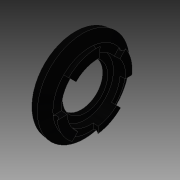
# Autodesk Inventor part: rope_pulley
Saved by Autodesk Inventor 2014 (Build 180170000, 170)
## iProperties
Created: 2013-12-08
Part Number: rope_pulley
Material: ABS Plastic
Document SubType Name: Modeling
Designer: buben
Density: 1.06 g/cm^3
Appearance: Anodized - Black
d0: 45,00 deg
d1: 1,000 mm
d2: 3,000 mm
d4: 6,000 mm
d5: 2,000 mm
d8: 7,000 mm
d9: 17,000 mm
d10: 22,000 mm
d12: 4,000 ul
d14: 135,00 deg
d16: 4,424 mm
d17: 0,00 deg
d18: 2,424 mm
d19: 0,00 deg
d20: 1,000 mm
Author: buben
Autodesk Inventor part; units mm, degrees
ref_plane "YZ Plane" through (0, 0, 0) normal (1, 0, 0) x (0, 1, 0)
ref_plane "XZ Plane" through (0, 0, 0) normal (0, 1, 0) x (-1, 0, 0)
ref_plane "XY Plane" through (0, 0, 0) normal (0, 0, 1) x (1, 0, 0)
sketch "Sketch1" plane through (0, 0, 0) normal (0, 0, 1) x (1, 0, 0)
  line L0 (3.175, 17) -> (4.5761, 13.6173)
  line L1 (6.4239, 13.6173) -> (7.825, 17)
  arc A0 (4.5761, 13.6173) -> (6.4239, 13.6173) centre (5.5, 14) ccw
  line L2 (7.825, 17) -> (9, 17)
  line L3 (3.175, 17) -> (0, 17)
  line L4 (2, 11) -> (9, 11)
  line L5 (9, 17) -> (9, 11)
  line L6 (0, 17) -> (0, 8.5)
  line L7 (2, 11) -> (2, 8.5)
  line L8 (2, 8.5) -> (0, 8.5)
  line L9 (0, 0) -> (2, 0) construction
  point P0 (5.5, 11)
  dimension "d0" = 45
  dimension "d1" = 1
  dimension "d2" = 3
  dimension "d4" = 6
  dimension "d5" = 2
  dimension "d8" = 7
  dimension "d9" = 17
  dimension "d10" = 22
  constraints: 20 end point, 4 parallel, 4 vertical alignment, 2 perpendicular, 2 point on circle, 2 tangent, 1 centre point, 1 coincident, 1 collinear, 1 equal length, 1 horizontal, 1 horizontal alignment, 1 midpoint
  measures "d0" angle of L1 L0
  measures "d1" radius of A0
  measures "d2" vertical distance of L0.start A0.centre
  measures "d4" distance of L4.end L2.end
  measures "d5" distance of L7.end L6.end
  measures "d8" distance of L4.start L4.end
  measures "d9" diameter of L8 L9
  measures "d10" diameter of L4 L9
revolve "Revolution1" add sketch "Sketch1" angle 360 about axis through (0, 0, 0) along (1, 0, 0)
sketch "Sketch2" plane through (9, 0, 0) normal (1, 0, 0) x (0, 0, -1)
  circle A0 centre (0, 0) radius 11 projected
  circle A1 centre (0, 0) radius 17 projected
  line L0 (-17, 0) -> (17, 0) construction
  line L1 (-12.0208, -12.0208) -> (12.0208, 12.0208) construction
  line L2 (0, -17) -> (0, 17) construction
  line L3 (12.0208, -12.0208) -> (-12.0208, 12.0208) construction
  line L4 (-17, 0) -> (-11, 0)
  line L5 (-7.7782, 7.7782) -> (-12.0208, 12.0208)
  line L6 (0, 17) -> (0, 11)
  line L7 (12.0208, 12.0208) -> (7.7782, 7.7782)
  line L8 (11, 0) -> (17, 0)
  line L9 (12.0208, -12.0208) -> (7.7782, -7.7782)
  line L10 (0, -17) -> (0, -11)
  line L11 (-7.7782, -7.7782) -> (-12.0208, -12.0208)
  arc A2 (7.7782, 7.7782) -> (0, 11) centre (0, 0) ccw
  arc A3 (12.0208, 12.0208) -> (0, 17) centre (0, 0) ccw
  arc A4 (7.7782, -7.7782) -> (11, 0) centre (0, 0) ccw
  arc A5 (12.0208, -12.0208) -> (17, 0) centre (0, 0) ccw
  arc A6 (-12.0208, 12.0208) -> (-17, 0) centre (0, 0) ccw
  arc A7 (-12.0208, -12.0208) -> (0, -17) centre (0, 0) ccw
  arc A8 (-7.7782, 7.7782) -> (-11, 0) centre (0, 0) ccw
  arc A9 (-7.7782, -7.7782) -> (0, -11) centre (0, 0) ccw
  dimension "d14" = 135
  constraints: 25 end point, 18 point on circle, 8 centre point, 8 point on line, 4 concentric, 4 midpoint, 3 coincident, 2 collinear, 1 horizontal, 12 other
extrude "Extrusion1" cut sketch "Sketch2" against normal blind 4.424 contours L8 A1 L9 A0 | A0 L6 A1 L7 | L10 A1 L11 A0 | A0 L4 A1 L5
sketch "Sketch3" plane through (9, 0, 17) normal (1, 0, 0) x (0, 0, -1)
  line L0 (4.9792, -12.0208) -> (9.2218, -7.7782) projected
  arc A0 (6, 0) -> (9.2218, -7.7782) centre (17, 0) ccw projected
  line L1 (6, 0) -> (0, 0) projected
  arc A1 (0, 0) -> (4.9792, -12.0208) centre (17, 0) ccw projected
  line L2 (4.9792, 12.0208) -> (9.2218, 7.7782) projected
  arc A2 (17, 11) -> (9.2218, 7.7782) centre (17, 0) ccw projected
  line L3 (17, 11) -> (17, 17) projected
  arc A3 (17, 17) -> (4.9792, 12.0208) centre (17, 0) ccw projected
  line L4 (28, 0) -> (34, 0) projected
  arc A4 (34, 0) -> (29.0208, 12.0208) centre (17, 0) ccw projected
  line L5 (29.0208, 12.0208) -> (24.7782, 7.7782) projected
  arc A5 (28, 0) -> (24.7782, 7.7782) centre (17, 0) ccw projected
  line L6 (17, -11) -> (17, -17) projected
  arc A6 (17, -17) -> (29.0208, -12.0208) centre (17, 0) ccw projected
  line L7 (29.0208, -12.0208) -> (24.7782, -7.7782) projected
  arc A7 (17, -11) -> (24.7782, -7.7782) centre (17, 0) ccw projected
extrude "Extrusion2" cut sketch "Sketch3" against normal blind 2.424
chamfer "Chamfer1" distance 1 angle 45 1 edges at (0, -17, 0)
body "Solid1"
